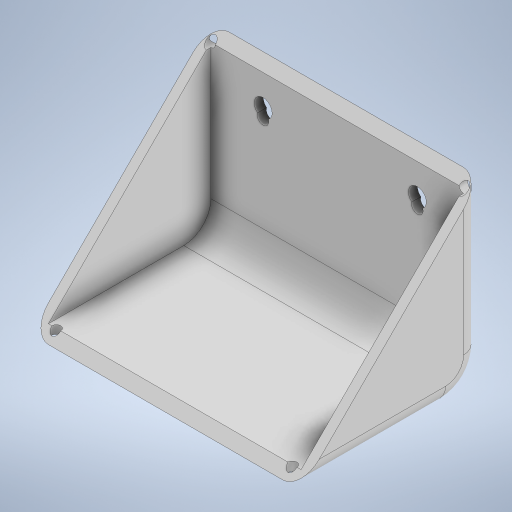
# Autodesk Inventor part: shell
Saved by Autodesk Inventor 2023 (Build 270158000, 158)
## iProperties
Created: 2023-02-11
Part Number: shell
Material: Generic
Document SubType Name: Modeling
Designer: Lauren
Density: 1 g/cm^3
Appearance: Default
Author: Lauren
Autodesk Inventor part; units mm, degrees
ref_plane "YZ Plane" through (0, 0, 0) normal (1, 0, 0) x (0, 1, 0)
ref_plane "XZ Plane" through (0, 0, 0) normal (0, 1, 0) x (-1, 0, 0)
ref_plane "XY Plane" through (0, 0, 0) normal (0, 0, 1) x (1, 0, 0)
sketch "Sketch1" plane through (0, 0, 0) normal (1, 0, 0) x (0, 1, 0)
  line L0 (0, 0) -> (127, 0)
  line L1 (0, 0) -> (0, 127)
  line L2 (0, 127) -> (127, 0)
  dimension "d0" = 127
  dimension "d1" = 127
  constraints: 6 end point, 1 horizontal, 1 vertical
  measures "d0" distance of L0.start L0.end
  measures "d1" distance of L0.start L1.end
extrude "Extrusion1" add sketch "Sketch1" along normal blind 190.5
fillet "Fillet1" radius 25.4 1 edges at (95.25, 0, 0)
shell "Shell1" thickness 6.35 removed faces 1 at (127, 84.6667, 42.3333)
fillet "Fillet2" radius 12.7 6 edges at (190.5, 7.4395, 7.4395) (190.5, 0, 76.2) (190.5, 76.2, 0) (0, 7.4395, 7.4395) (0, 0, 76.2) (0, 76.2, 0)
sketch "Sketch2" plane through (177.8, 127, 0) normal (0, 0, -1) x (-1, 0, 0)
  line L0 (7.0063, -88.7561) -> (13.3563, -88.7561)
  line L1 (13.3563, -88.7561) -> (13.3563, -152.2561)
  line L2 (13.3563, -152.2561) -> (7.0063, -152.2561)
  line L3 (7.0063, -152.2561) -> (7.0063, -88.7561)
  point P0 (177.8, -127)
  dimension "d7" = 6.35
  dimension "d8" = 63.5
  constraints: 8 end point, 2 parallel, 1 horizontal, 1 perpendicular
  measures "d7" distance of L1.end L2.end
  measures "d8" distance of L0.end L1.end
extrude "Extrusion2" cut sketch "Sketch2" against normal blind 25.4
sketch "Sketch3" plane through (177.8, 127, 0) normal (0, 0, -1) x (-1, 0, 0)
  circle A0 centre (26.2137, -27.9058) radius 6.35
  circle A1 centre (134.6629, -27.9058) radius 6.35
  point P0 (177.8, -127)
  dimension "d11" = 12.7
  dimension "d12" = 12.7
  constraints: 2 centre point
  measures "d11" diameter of A0
  measures "d12" diameter of A1
extrude "Extrusion3" cut sketch "Sketch3" against normal blind 25.4
sketch "Sketch4" plane through (177.8, 127, 0) normal (0, 0, -1) x (-1, 0, 0)
  circle A0 centre (26.2137, -27.9058) radius 6.35 projected
  circle A1 centre (26.2137, -34.2558) radius 4.1275
  circle A2 centre (134.749, -34.2558) radius 4.1275
  point P0 (177.8, -127)
  dimension "d15" = 8.255
  dimension "d16" = 8.255
  constraints: 2 centre point, 1 vertical alignment, 1 other
  measures "d15" diameter of A1
  measures "d16" diameter of A2
extrude "Extrusion4" cut sketch "Sketch4" against normal blind 25.4 contours A1 A0 | A0 A1 | A2 picked at (25.4127, -32.8707) picked at (27.1236, -35.5058)
sketch "Sketch5" plane through (177.8, 127, 0) normal (0, 0, -1) x (-1, 0, 0)
  point P0 (177.8, -127)
  point P1 (-6.35, -6.35)
  point P2 (171.45, -6.35)
  point P3 (171.45, -6.35)
  constraints: 1 coincident
hole "Hole1" at (184.15, 120.65, 0) at (6.35, 120.65, 0) direction (0, 0, 1) diameter 6.35 end through all
sketch "Sketch6" plane through (12.7, 0, 127) normal (0, -1, 0) x (1, 0, 0)
  line L0 (171.45, -6.35) -> (-6.35, -6.35) projected
  point P0 (-12.7, -127)
  point P1 (-0.7443, -6.35)
  point P2 (165.3424, -6.35)
  constraints: 2 point on line
hole "Hole2" at (11.9557, 0, 120.65) at (178.0424, 0, 120.65) direction (0, 1, 0) diameter 6.35 end through all
body "Solid1"
